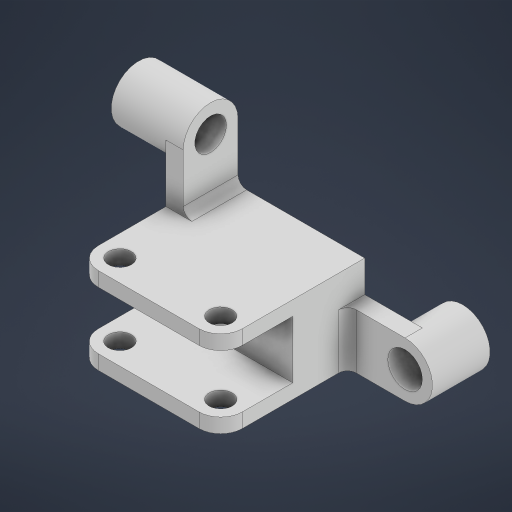
# Autodesk Inventor part: Część24
Saved by Autodesk Inventor 2023 (Build 270158000, 158)
## iProperties
Created: 2023-05-09
Part Number: Część24
Material: Ogólny
Document SubType Name: Modeling
Designer: Adam
Density: 1 g/cm^3
Appearance: Domyślna
Author: Adam
Autodesk Inventor part; units mm, degrees
ref_plane "YZ Plane" through (0, 0, 0) normal (1, 0, 0) x (0, 1, 0)
ref_plane "XZ Plane" through (0, 0, 0) normal (0, 1, 0) x (-1, 0, 0)
ref_plane "XY Plane" through (0, 0, 0) normal (0, 0, 1) x (1, 0, 0)
sketch "Szkic1" plane through (0, 0, 0) normal (0, 1, 0) x (-1, 0, 0)
  line L0 (-15, 0) -> (-85, 0)
  line L1 (-100, -15) -> (-100, -100)
  line L2 (-100, -100) -> (0, -100)
  line L3 (0, -100) -> (0, -15)
  arc A0 (0, -15) -> (-15, 0) centre (-15, -15) ccw
  arc A1 (-85, 0) -> (-100, -15) centre (-85, -15) ccw
  point P0 (0, 0)
  point P1 (-100, 0)
  dimension "d0" = 100
  dimension "d1" = 100
  dimension "d2" = 15
  constraints: 8 end point, 4 point on circle, 4 point on line, 4 tangent, 2 centre point, 2 parallel, 1 equal radius, 1 horizontal, 1 perpendicular
  measures "d0" distance of L2.end L1.end
  measures "d1" distance of L1.end point (-100, 0)
  measures "d2" radius of A0
extrude "Wyciągnięcie proste1" add sketch "Szkic1" along normal blind 10
sketch "Szkic2" plane through (0, 10, 0) normal (0, 1, 0) x (1, 0, 0)
  line L0 (0, 100) -> (100, 100)
  line L1 (100, 100) -> (100, 50)
  line L2 (100, 50) -> (0, 50)
  line L3 (0, 50) -> (0, 100)
  point P0 (0, 0)
  dimension "d5" = 100
  dimension "d6" = 50
  constraints: 8 end point, 2 parallel, 1 horizontal, 1 perpendicular
  measures "d5" distance of L1.end L2.end
  measures "d6" distance of L0.end L1.end
extrude "Wyciągnięcie proste2" add sketch "Szkic2" along normal blind 20
sketch "Szkic3" plane through (0, 10, 0) normal (0, 1, 0) x (1, 0, 0)
  arc A0 (0, 15) -> (15, 0) centre (15, 15) ccw projected
  arc A1 (85, 0) -> (100, 15) centre (85, 15) ccw projected
  point P0 (0, 0)
  constraints: 2 coincident
hole "Otwór1" at (15, 10, -15) at (85, 10, -15) direction (0, -1, 0) diameter 16 end through all
mirror "Odbij1" about plane through (50, 30, -75) normal (0, 1, 0) of "Wyciągnięcie proste1", "Otwór1", "Wyciągnięcie proste2"
sketch "Szkic4" plane through (100, 0, -100) normal (0, 0, -1) x (-1, 0, 0)
  circle A0 centre (-40, 19) radius 19
  line L0 (15, 0) -> (0, 0) projected
  line L1 (0, 0) -> (-40, 0)
  line L2 (-40, 38) -> (0, 38)
  line L3 (0, 10) -> (0, 50) projected
  line L4 (0, 0) -> (0, 38)
  point P0 (100, 0)
  dimension "d16" = 38
  dimension "d17" = 40
  constraints: 6 end point, 2 horizontal, 2 point on circle, 1 centre point, 1 point on line, 1 tangent, 1 vertical
  measures "d16" diameter of A0
  measures "d17" distance of L0.end L1.end
extrude "Wyciągnięcie proste3" add sketch "Szkic4" against normal blind 12
sketch "Szkic5" plane through (100, 60, -100) normal (0, 0, -1) x (-1, 0, 0)
  arc A0 (-40, -22) -> (-40, -60) centre (-40, -41) ccw projected
  circle A1 centre (-40, -41) radius 19
  point P0 (100, -60)
  point P1 (-40, -22)
  dimension "d20" = 38
  constraints: 1 centre point, 1 coincident
  measures "d20" diameter of A1
extrude "Wyciągnięcie proste4" add sketch "Szkic5" along normal blind 28
sketch "Szkic6" plane through (140, 19, -128) normal (0, 0, -1) x (-1, 0, 0)
  point P0 (140, -19)
  point P1 (0, 0)
hole "Otwór2" at (140, 19, -128) direction (0, 0, 1) diameter 24 end through all
fillet "Zaokrąglenie1" radius 6 1 edges at (100, 19, -88)
sketch "Szkic7" plane through (0, 0, -100) normal (-1, 0, 0) x (0, 0, 1)
  circle A0 centre (19, 100) radius 19
  line L0 (0, 0) -> (0, 60) projected
  line L1 (0, 60) -> (0, 100)
  line L2 (38, 100) -> (38, 60)
  line L3 (0, 60) -> (85, 60) projected
  point P0 (100, 0)
  dimension "d31" = 38
  dimension "d32" = 40
  constraints: 4 end point, 2 point on circle, 2 vertical, 1 centre point, 1 point on line, 1 tangent
  measures "d31" diameter of A0
  measures "d32" distance of L0.end L1.end
extrude "Wyciągnięcie proste5" add sketch "Szkic7" against normal blind 12
sketch "Szkic8" plane through (0, 0, -100) normal (-1, 0, 0) x (0, 0, 1)
  arc A0 (38, 100) -> (0, 100) centre (19, 100) ccw projected
  circle A1 centre (19, 100) radius 19
  point P0 (100, 0)
  dimension "d35" = 38
  constraints: 1 centre point, 1 coincident
  measures "d35" diameter of A1
extrude "Wyciągnięcie proste6" add sketch "Szkic8" along normal blind 38
sketch "Szkic9" plane through (-38, 100, -81) normal (-1, 0, 0) x (0, 0, 1)
  point P0 (81, -100)
  point P1 (0, 0)
hole "Otwór3" at (-38, 100, -81) direction (1, 0, 0) diameter 22 end through all
fillet "Zaokrąglenie2" radius 6 1 edges at (12, 60, -81)
